# Autodesk Inventor part: 787
Saved by Autodesk Inventor 2015 SP1 (Build 190203100, 203)
## iProperties
Created: 2015-10-19
Part Number: 787
Material: Generic
Document SubType Name: Modeling
Designer: Kartikye
Density: 1 g/cm^3
Appearance: R0805, 787
Author: Kartikye
Autodesk Inventor part; units mm, degrees
ref_plane "YZ Plane" through (0, 0, 0) normal (1, 0, 0) x (0, 1, 0)
ref_plane "XZ Plane" through (0, 0, 0) normal (0, 1, 0) x (-1, 0, 0)
ref_plane "XY Plane" through (0, 0, 0) normal (0, 0, 1) x (1, 0, 0)
sketch "R0805, 787_69" plane through (0, 0, 0) normal (0, 0, 1) x (1, 0, 0)
  line L0 (-1.973, 0.983) -> (1.973, 0.983)
  line L1 (1.973, 0.983) -> (1.973, -0.983)
  line L2 (1.973, -0.983) -> (-1.973, -0.983)
  line L3 (-1.973, -0.983) -> (-1.973, 0.983)
  constraints: 8 end point
extrude "Extrusion1" add sketch "R0805, 787_69" along normal blind 1
body "Solid1"
